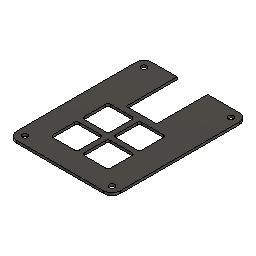
Lid (Autodesk Fusion 360 design; units mm, degrees)
Autodesk Fusion 360 part; units mm, degrees
note: some values were not read from the file. Set by a fixed rule: which face or edge a step refers to.
sketch "plate-2025-12-08T19_56_41.367Z" plane through (0, 0, 0) normal (0, 0, 1) x (1, 0, 0)
  line L0 (3.025, -2.525) -> (16.025, -2.525)
  line L1 (3.025, -16.525) -> (16.025, -16.525)
  line L2 (2.525, -3.025) -> (2.525, -16.025)
  line L3 (16.525, -3.025) -> (16.525, -16.025)
  arc A0 (3.025, -2.525) -> (2.525, -3.025) centre (3.025, -3.025) ccw
  arc A1 (16.525, -3.025) -> (16.025, -2.525) centre (16.025, -3.025) ccw
  arc A2 (2.525, -16.025) -> (3.025, -16.525) centre (3.025, -16.025) ccw
  arc A3 (16.025, -16.525) -> (16.525, -16.025) centre (16.025, -16.025) ccw
  line L4 (22.075, -2.525) -> (35.075, -2.525)
  line L5 (22.075, -16.525) -> (35.075, -16.525)
  line L6 (21.575, -3.025) -> (21.575, -16.025)
  line L7 (35.575, -3.025) -> (35.575, -16.025)
  arc A4 (22.075, -2.525) -> (21.575, -3.025) centre (22.075, -3.025) ccw
  arc A5 (35.575, -3.025) -> (35.075, -2.525) centre (35.075, -3.025) ccw
  arc A6 (21.575, -16.025) -> (22.075, -16.525) centre (22.075, -16.025) ccw
  arc A7 (35.075, -16.525) -> (35.575, -16.025) centre (35.075, -16.025) ccw
  line L8 (3.025, -21.575) -> (16.025, -21.575)
  line L9 (3.025, -35.575) -> (16.025, -35.575)
  line L10 (2.525, -22.075) -> (2.525, -35.075)
  line L11 (16.525, -22.075) -> (16.525, -35.075)
  arc A8 (3.025, -21.575) -> (2.525, -22.075) centre (3.025, -22.075) ccw
  arc A9 (16.525, -22.075) -> (16.025, -21.575) centre (16.025, -22.075) ccw
  arc A10 (2.525, -35.075) -> (3.025, -35.575) centre (3.025, -35.075) ccw
  arc A11 (16.025, -35.575) -> (16.525, -35.075) centre (16.025, -35.075) ccw
  line L12 (22.075, -21.575) -> (35.075, -21.575)
  line L13 (22.075, -35.575) -> (35.075, -35.575)
  line L14 (21.575, -22.075) -> (21.575, -35.075)
  line L15 (35.575, -22.075) -> (35.575, -35.075)
  arc A12 (22.075, -21.575) -> (21.575, -22.075) centre (22.075, -22.075) ccw
  arc A13 (35.575, -22.075) -> (35.075, -21.575) centre (35.075, -22.075) ccw
  arc A14 (21.575, -35.075) -> (22.075, -35.575) centre (22.075, -35.075) ccw
  arc A15 (35.075, -35.575) -> (35.575, -35.075) centre (35.075, -35.075) ccw
  line L16 (-11.42, 33.161) -> (51.48, 33.161)
  line L17 (51.48, 33.161) -> (51.48, -49.139)
  line L18 (51.48, -49.139) -> (-11.42, -49.139)
  line L19 (-11.42, -49.139) -> (-11.42, 33.161)
  circle A16 centre (-6.42, -44.139) radius 1.7
  circle A17 centre (46.48, -44.139) radius 1.7
  circle A18 centre (-6.42, 28.161) radius 1.7
  circle A19 centre (46.48, 28.161) radius 1.7
  line L20 (8.79, 33.161) -> (27.29, 33.161)
  line L21 (27.29, 33.161) -> (27.29, 2.161)
  line L22 (27.29, 2.161) -> (8.79, 2.161)
  line L23 (8.79, 2.161) -> (8.79, 33.161)
  line L24 (3.525, -22.575) -> (15.525, -22.575)
  line L25 (15.525, -22.575) -> (15.525, -34.575)
  line L26 (3.525, -34.575) -> (15.525, -34.575)
  line L27 (3.525, -22.575) -> (3.525, -34.575)
  line L28 (1.525, -3.025) -> (1.525, -16.025)
  arc A20 (1.525, -16.025) -> (3.025, -17.525) centre (3.025, -16.025) ccw
  line L29 (3.025, -17.525) -> (16.025, -17.525)
  arc A21 (16.025, -17.525) -> (17.525, -16.025) centre (16.025, -16.025) ccw
  line L30 (17.525, -3.025) -> (17.525, -16.025)
  arc A22 (17.525, -3.025) -> (16.025, -1.525) centre (16.025, -3.025) ccw
  line L31 (3.025, -1.525) -> (16.025, -1.525)
  arc A23 (3.025, -1.525) -> (1.525, -3.025) centre (3.025, -3.025) ccw
  line L32 (34.575, -22.575) -> (34.575, -34.575)
  line L33 (22.575, -34.575) -> (34.575, -34.575)
  line L34 (22.575, -22.575) -> (22.575, -34.575)
  line L35 (22.575, -22.575) -> (34.575, -22.575)
  arc A24 (22.075, -1.525) -> (20.575, -3.025) centre (22.075, -3.025) ccw
  line L36 (20.575, -3.025) -> (20.575, -16.025)
  arc A25 (20.575, -16.025) -> (22.075, -17.525) centre (22.075, -16.025) ccw
  line L37 (22.075, -17.525) -> (35.075, -17.525)
  arc A26 (35.075, -17.525) -> (36.575, -16.025) centre (35.075, -16.025) ccw
  line L38 (36.575, -3.025) -> (36.575, -16.025)
  arc A27 (36.575, -3.025) -> (35.075, -1.525) centre (35.075, -3.025) ccw
  line L39 (22.075, -1.525) -> (35.075, -1.525)
  line L40 (20.575, -22.075) -> (20.575, -35.075)
  arc A28 (20.575, -35.075) -> (22.075, -36.575) centre (22.075, -35.075) ccw
  line L41 (22.075, -36.575) -> (35.075, -36.575)
  arc A29 (35.075, -36.575) -> (36.575, -35.075) centre (35.075, -35.075) ccw
  line L42 (36.575, -22.075) -> (36.575, -35.075)
  arc A30 (36.575, -22.075) -> (35.075, -20.575) centre (35.075, -22.075) ccw
  line L43 (22.075, -20.575) -> (35.075, -20.575)
  arc A31 (22.075, -20.575) -> (20.575, -22.075) centre (22.075, -22.075) ccw
  arc A32 (3.025, -20.575) -> (1.525, -22.075) centre (3.025, -22.075) ccw
  line L44 (1.525, -22.075) -> (1.525, -35.075)
  arc A33 (1.525, -35.075) -> (3.025, -36.575) centre (3.025, -35.075) ccw
  line L45 (3.025, -36.575) -> (16.025, -36.575)
  arc A34 (16.025, -36.575) -> (17.525, -35.075) centre (16.025, -35.075) ccw
  line L46 (17.525, -22.075) -> (17.525, -35.075)
  arc A35 (17.525, -22.075) -> (16.025, -20.575) centre (16.025, -22.075) ccw
  line L47 (3.025, -20.575) -> (16.025, -20.575)
  dimension "d1" = 82.3
  dimension "d2" = 62.9
  dimension "d3" = 13.564
  dimension "d5" = 13.945
  dimension "d6" = 3.4
  dimension "d7" = 3.4
  dimension "d8" = 3.4
  dimension "d9" = 3.4
  dimension "d10" = 18.5
  dimension "d11" = 31
  dimension "d12" = 5
  dimension "d13" = 5
  dimension "d14" = 5
  dimension "d15" = 5
  dimension "d16" = 5
  dimension "d17" = 5
  dimension "d18" = 5
  dimension "d19" = 5
  dimension "d20" = 20.21
  dimension "d33" = 1
  dimension "d34" = 1
  dimension "d35" = 1
  constraint horizontal L16
  constraint vertical L17
  constraint horizontal L18
  constraint vertical L19
  constraint horizontal L20
  constraint vertical L21
  constraint horizontal L22
  constraint vertical L23
  constraint coincident L16 L20.start
  measures "d1" distance of L16.start L18.end
  measures "d2" distance of L16.start L16.end
  measures "d3" distance of L9 L18
  measures "d5" distance of L10 L19
  measures "d6" diameter of A16
  measures "d7" diameter of A17
  measures "d8" diameter of A18
  measures "d9" diameter of A19
  measures "d10" distance of L20.start L20.end
  measures "d11" distance of L20.start L22.end
  measures "d12" distance of L16 A18.centre
  measures "d13" distance of L16 A19.centre
  measures "d14" distance of L19 A18.centre
  measures "d15" distance of L17 A19.centre
  measures "d16" distance of L18 A17.centre
  measures "d17" distance of L17 A17.centre
  measures "d18" distance of L18 A16.centre
  measures "d19" distance of L19 A16.centre
  measures "d20" distance of L19 L23
  measures "d34" distance of A13
  measures "d35" distance of A11
extrude "Extrude1" add sketch "plate-2025-12-08T19_56_41.367Z" along normal blind 1.5 contours L16 L17 L18 L19 L21 L22 L23
fillet "Fillet1" radius 5 2 edges at (51.48, -49.139, 0.75) (-11.42, -49.139, 0.75)
fillet "Fillet2" radius 5 2 edges at (51.48, 33.161, 0.75) (-11.42, 33.161, 0.75)
sketch "Sketch2" plane through (0, 0, 0) normal (0, 0, -1) x (1, 0, 0)
  circle A0 centre (-6.42, 44.139) radius 1.7
  circle A1 centre (46.48, 44.139) radius 1.7
  circle A2 centre (-6.42, -28.161) radius 1.7
  circle A3 centre (46.48, -28.161) radius 1.7
  arc A4 (-11.42, -28.161) -> (-6.42, -33.161) centre (-6.42, -28.161) ccw
  line L0 (-6.42, -33.161) -> (8.79, -33.161)
  line L1 (8.79, -33.161) -> (8.79, -2.161)
  line L2 (8.79, -2.161) -> (27.29, -2.161)
  line L3 (27.29, -2.161) -> (27.29, -33.161)
  line L4 (27.29, -33.161) -> (46.48, -33.161)
  arc A5 (46.48, -33.161) -> (51.48, -28.161) centre (46.48, -28.161) ccw
  line L5 (51.48, -28.161) -> (51.48, 44.139)
  arc A6 (51.48, 44.139) -> (46.48, 49.139) centre (46.48, 44.139) ccw
  line L6 (46.48, 49.139) -> (-6.42, 49.139)
  arc A7 (-6.42, 49.139) -> (-11.42, 44.139) centre (-6.42, 44.139) ccw
  line L7 (-11.42, 44.139) -> (-11.42, -28.161)
  line L8 (0, 40) -> (20, 40) construction
  line L9 (20, 40) -> (20, 45) construction
  line L10 (20, 45) -> (0, 45) construction
  line L11 (0, 45) -> (0, 40) construction
  arc A8 (16.025, 1.525) -> (17.525, 3.025) centre (16.025, 3.025) ccw
  line L12 (16.025, 1.525) -> (3.025, 1.525)
  arc A9 (1.525, 3.025) -> (3.025, 1.525) centre (3.025, 3.025) ccw
  line L13 (1.525, 3.025) -> (1.525, 16.025)
  arc A10 (3.025, 17.525) -> (1.525, 16.025) centre (3.025, 16.025) ccw
  line L14 (3.025, 17.525) -> (16.025, 17.525)
  arc A11 (17.525, 16.025) -> (16.025, 17.525) centre (16.025, 16.025) ccw
  line L15 (17.525, 16.025) -> (17.525, 3.025)
  line L16 (20.575, 3.025) -> (20.575, 16.025)
  arc A12 (22.075, 17.525) -> (20.575, 16.025) centre (22.075, 16.025) ccw
  line L17 (22.075, 17.525) -> (35.075, 17.525)
  arc A13 (36.575, 16.025) -> (35.075, 17.525) centre (35.075, 16.025) ccw
  line L18 (36.575, 16.025) -> (36.575, 3.025)
  arc A14 (35.075, 1.525) -> (36.575, 3.025) centre (35.075, 3.025) ccw
  line L19 (35.075, 1.525) -> (22.075, 1.525)
  arc A15 (20.575, 3.025) -> (22.075, 1.525) centre (22.075, 3.025) ccw
  line L20 (1.525, 22.075) -> (1.525, 35.075)
  arc A16 (3.025, 36.575) -> (1.525, 35.075) centre (3.025, 35.075) ccw
  line L21 (3.025, 36.575) -> (16.025, 36.575)
  arc A17 (17.525, 35.075) -> (16.025, 36.575) centre (16.025, 35.075) ccw
  line L22 (17.525, 35.075) -> (17.525, 22.075)
  arc A18 (16.025, 20.575) -> (17.525, 22.075) centre (16.025, 22.075) ccw
  line L23 (16.025, 20.575) -> (3.025, 20.575)
  arc A19 (1.525, 22.075) -> (3.025, 20.575) centre (3.025, 22.075) ccw
  arc A20 (35.075, 20.575) -> (36.575, 22.075) centre (35.075, 22.075) ccw
  line L24 (35.075, 20.575) -> (22.075, 20.575)
  arc A21 (20.575, 22.075) -> (22.075, 20.575) centre (22.075, 22.075) ccw
  line L25 (20.575, 22.075) -> (20.575, 35.075)
  arc A22 (22.075, 36.575) -> (20.575, 35.075) centre (22.075, 35.075) ccw
  line L26 (22.075, 36.575) -> (35.075, 36.575)
  arc A23 (36.575, 35.075) -> (35.075, 36.575) centre (35.075, 35.075) ccw
  line L27 (36.575, 35.075) -> (36.575, 22.075)
  dimension "d27" = 2
  text T0 "Ángel\"s Hackpad" font "Arial" height 2 align left top in box 20 x 5 at (0, 40) x (1, 0) y (0, 1) spacing 1 kerned
extrude "Extrude2" cut sketch "Sketch2" against normal blind 0.2 text T0
extrude "Extrude3" add 1 faces at (7.3943, -44.5457, 0.2) along direction (0, 0, -1) blind 0.2
equation "d3 = 9.5 mm + 4.064 mm"
equation "d5 = 9.5 mm + 4.445 mm"
equation "d20 = 14.46 mm + 5.75 mm"
equation "d28 = 'Ángel\"s Hackpad'"
named bodies: "Lid"
